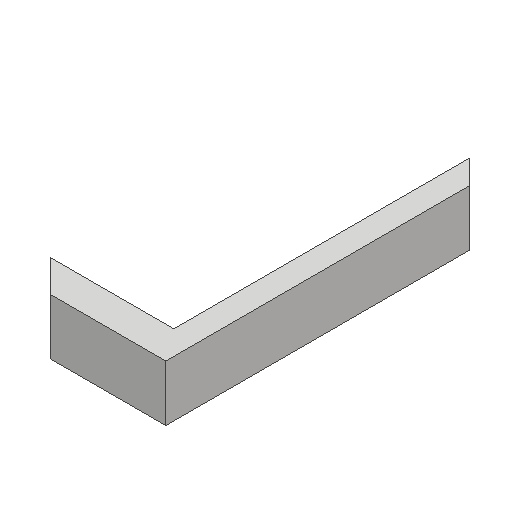
# Autodesk Inventor part: 3DP_PLA_Front_motor_clamp_hole_plug
Saved by Autodesk Inventor 2026.1 (Build 301233000, 233)
## iProperties
Created: 2016-05-02
Part Number: 3DP_PLA_Front_motor_clamp_hole_plug
Material: Ogólny
Document SubType Name: Modeling
Designer: Andrzej
Density: 1 g/cm^3
Appearance: Domyślna
Mass: 1.16585 g
Surface Area: 11.1665 cm^2
Volume: 1.16585 cm^3
Author: Andrzej
Autodesk Inventor part; units mm, degrees
ref_plane "YZ Plane" through (0, 0, 0) normal (1, 0, 0) x (0, 1, 0)
ref_plane "XZ Plane" through (0, 0, 0) normal (0, 1, 0) x (-1, 0, 0)
ref_plane "XY Plane" through (0, 0, 0) normal (0, 0, 1) x (1, 0, 0)
sketch "Szkic1" plane through (0, 0, 0) normal (0, 0, 1) x (1, 0, 0)
  line L0 (-6.6672, -2.767) -> (7.8328, -2.767)
  line L1 (7.8328, -2.767) -> (7.8328, 35.333)
  line L2 (7.8328, 35.333) -> (4.8328, 35.333)
  line L3 (4.8328, 35.333) -> (4.8328, 1.233)
  line L4 (4.8328, 1.233) -> (-6.6672, 1.233)
  line L5 (-6.6672, 1.233) -> (-6.6672, -2.767)
  point P0 (0, 0)
  dimension "d0" = 14.5
  dimension "d1" = 38.1
  dimension "d3" = 34.1
  dimension "d8" = 3
  constraints: 12 end point, 4 perpendicular, 1 horizontal, 1 vertical
  measures "d0" distance of L0.start L0.end
  measures "d1" distance of L0.end L1.end
  measures "d3" distance of L2.end L3.end
  measures "d8" distance between parallel lines of L1 L3
extrude "Wyciągnięcie proste1" add sketch "Szkic1" along normal blind 7
sketch "Szkic2" plane through (0, 0, 7) normal (0, 0, 1) x (1, 0, 0)
  line L0 (-6.6672, -2.767) -> (7.8328, -2.767) projected
  line L1 (7.8328, -2.767) -> (7.8328, 35.333) projected
  line L2 (7.8328, 35.333) -> (4.8328, 35.333) projected
  line L3 (4.8328, 35.333) -> (4.8328, 1.233) projected
  line L4 (4.8328, 1.233) -> (-6.6672, 1.233) projected
  line L5 (-6.6672, 1.233) -> (-6.6672, -2.767) projected
  line L6 (-6.6672, -2.767) -> (-10.6672, 1.233)
  line L7 (-6.6672, -2.767) -> (1.7978, -2.767) construction
  line L8 (-6.6672, 1.233) -> (-6.6672, -2.767)
  line L9 (4.8328, 1.233) -> (-6.6672, 1.233) projected
  line L10 (-6.6672, 1.233) -> (-10.6672, 1.233)
  line L11 (7.8328, 35.333) -> (4.8328, 35.333) projected
  line L12 (7.8328, 35.333) -> (4.8328, 38.333)
  line L13 (7.8328, 35.333) -> (13.4348, 35.333) construction
  line L14 (4.8328, 35.333) -> (4.8328, 38.333)
  line L15 (4.8328, 35.333) -> (7.8328, 35.333)
  point P0 (0, 0)
  dimension "d12" = 135
  dimension "d14" = 135
  constraints: 16 end point, 2 collinear, 2 horizontal, 2 vertical
  measures "d12" angle of L7 L6
  measures "d14" angle of L13 L12
extrude "Wyciągnięcie proste2" add sketch "Szkic2" against normal blind 3.5 contours L6 L10 L5 | L2 L14 L12
